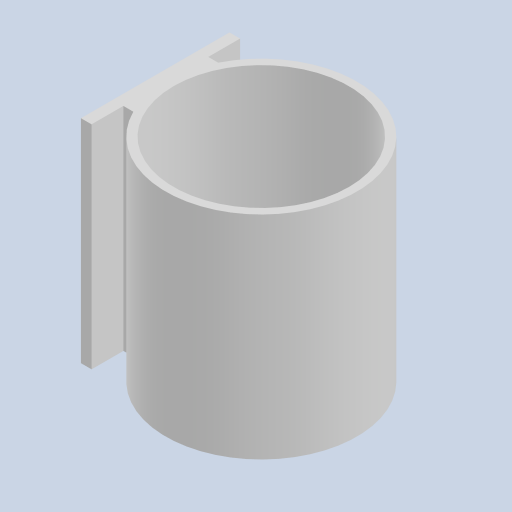
# Autodesk Inventor part: Part8
Saved by Autodesk Inventor 2024 (Build 280153000, 153)
## iProperties
Created: 2024-05-29
Part Number: Part8
Material: Generic
Document SubType Name: Modeling
Designer: mirun
Density: 1 g/cm^3
Appearance: Default
Author: mirun
Autodesk Inventor part; units mm, degrees
ref_plane "YZ Plane" through (0, 0, 0) normal (1, 0, 0) x (0, 1, 0)
ref_plane "XZ Plane" through (0, 0, 0) normal (0, 1, 0) x (-1, 0, 0)
sketch "Sketch1" plane through (0, 0, 0) normal (0, 1, 0) x (-1, 0, 0)
  circle A0 centre (0, 0) radius 16.5
  circle A1 centre (0, 0) radius 18
  dimension "d0" = 33
  dimension "d1" = 36
  constraints: 2 centre point, 2 coincident
  measures "d0" diameter of A0
  measures "d1" diameter of A1
extrude "Extrusion1" add sketch "Sketch1" along normal blind 40
sketch "Sketch2" plane through (0, 40, 0) normal (0, 1, 0) x (1, 0, 0)
  circle A0 centre (0, 0) radius 18 construction
  circle A1 centre (0, 0) radius 16.5 construction
  line L0 (0, 0) -> (-18, 0) construction
  constraints: 2 end point, 1 coincident, 1 horizontal, 1 horizontal alignment, 1 other
ref_plane "Work Plane1" through (-18, 40, 0) normal (-1, 0, 0) x (0, -1, 0)
sketch "Sketch3" plane through (-18, 40, 0) normal (-1, 0, 0) x (0, -1, 0)
  line L0 (0, 18) -> (0, -18) construction
  line L1 (40, 18) -> (40, -18) construction
  line L2 (0, 0) -> (40, 0)
  line L3 (40, 0) -> (40, -8)
  line L4 (40, -8) -> (0, -8)
  line L5 (0, -8) -> (0, 0)
  line L6 (40, 0) -> (40, 8)
  line L7 (40, 8) -> (0, 8)
  line L8 (0, 8) -> (0, 0)
  line L9 (0, -8) -> (40, -8)
  line L10 (40, -8) -> (40, -14)
  line L11 (40, -14) -> (0, -14)
  line L12 (0, -14) -> (0, -8)
  line L13 (0, 8) -> (40, 8)
  line L14 (40, 8) -> (40, 14)
  line L15 (40, 14) -> (0, 14)
  line L16 (0, 14) -> (0, 8)
  dimension "d4" = 8
  dimension "d5" = 6
  dimension "d6" = 6
  constraints: 30 end point, 6 parallel, 3 horizontal, 3 perpendicular, 3 point on line, 2 symmetric about line, 1 midpoint
  measures "d4" distance of L2.end L3.end
  measures "d5" distance of L9.end L10.end
  measures "d6" distance of L14.end L13.end
extrude "Extrusion2" add sketch "Sketch3" against normal up to surface contours L8 L7 L6 L2 | L2 L3 L4 L5
extrude "Extrusion3" add sketch "Sketch3" along normal blind 1
sketch "Sketch4" plane through (-19, 40, 0) normal (-1, 0, 0) x (0, 0, 1)
  line L0 (14, 0) -> (-14, 0) construction
  line L1 (-14, -40) -> (-10, -40)
  line L2 (-10, -40) -> (-10, 0)
  line L3 (-10, 0) -> (-14, 0)
  line L4 (-14, 0) -> (-14, -40)
  line L5 (-10, 0) -> (10.2529, 0)
  line L6 (10.2529, 0) -> (10.2529, -4)
  line L7 (10.2529, -4) -> (-10, -4)
  line L8 (-10, -4) -> (-10, 0)
  line L9 (14, -40) -> (10, -40)
  line L10 (10, -40) -> (10, 0)
  line L11 (10, 0) -> (14, 0)
  line L12 (14, 0) -> (14, -40)
  line L13 (10, -40) -> (-10, -40)
  line L14 (-10, -40) -> (-10, -36)
  line L15 (-10, -36) -> (10, -36)
  line L16 (10, -36) -> (10, -40)
  point P0 (0, -40)
  point P1 (10, -4)
  point P2 (-10, -4)
  dimension "d11" = 4
  dimension "d12" = 4
  dimension "d13" = 4
  dimension "d14" = 4
  constraints: 32 end point, 8 parallel, 4 horizontal, 4 perpendicular, 3 point on line
  measures "d11" distance of L3.end L2.end
  measures "d12" distance of L5.end L6.end
  measures "d13" distance of L10.end L11.end
  measures "d14" distance of L13.end L14.end
extrude "Extrusion4" add sketch "Sketch4" along normal blind 1 contours L4 L3 L2 L1 | L2 L15 L10 L13 | L10 L7 L6 L11 L12 L9 | L5 L10 L7 L2 | L5 L6 L7 L10
body "Solid1"
